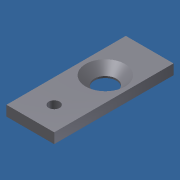
# Autodesk Inventor part: SUPORTE(44)
Saved by Autodesk Inventor 2012 SP1 (Build 160190100, 190)
## iProperties
Created: 2012-07-23
Part Number: SUPORTE(44)
Material: Carbon Steel
Document SubType Name: Modeling
Designer: bruno.silveira
Mass: 11.5689 g
Surface Area: 12.74 cm^2
Volume: 1.47 cm^3
Density: 7.87 g/cm^3
Author: bruno.silveira
Autodesk Inventor part; units mm, degrees
ref_plane "YZ Plane" through (0, 0, 0) normal (1, 0, 0) x (0, 1, 0)
ref_plane "XZ Plane" through (0, 0, 0) normal (0, 1, 0) x (-1, 0, 0)
ref_plane "XY Plane" through (0, 0, 0) normal (0, 0, 1) x (1, 0, 0)
sketch "Sketch1" plane through (0, 0, 0) normal (0, 0, 1) x (1, 0, 0)
  line L0 (0, 0) -> (14, 0)
  line L1 (14, 0) -> (14, 35)
  line L2 (14, 35) -> (0, 35)
  line L3 (0, 35) -> (0, 0)
  dimension "d0" = 14
  dimension "d1" = 35
  constraints: 8 end point, 2 parallel, 1 horizontal, 1 perpendicular
  measures "d0" distance of L1.end L2.end
  measures "d1" distance of L2.end L0.start
extrude "Extrusion1" add sketch "Sketch1" along normal blind 3
sketch "Sketch2" plane through (0, 0, 3) normal (0, 0, 1) x (1, 0, 0)
  line L0 (0, 0) -> (0, 35) projected
  line L1 (0, 35) -> (14, 35) projected
  point P0 (7, 22)
  dimension "d4" = 13
  dimension "d5" = 7
  measures "d4" distance from line of L1 point (7, 22)
  measures "d5" distance from line of L0 point (7, 22)
hole "Hole1" at (7, 22, 3) direction (0, 0, -1) diameter 6.5 depth 3 tip angle 118 countersink diameter 11.5 countersink angle 90
sketch "Sketch3" plane through (0, 0, 0) normal (0, 0, -1) x (-1, 0, 0)
  line L0 (0, 0) -> (-14, 0) projected
  line L1 (0, 35) -> (0, 0) projected
  point P0 (-7, 7)
  dimension "d13" = 7
  dimension "d14" = 7
  measures "d13" distance from line of L0 point (-7, 7)
  measures "d14" distance from line of L1 point (-7, 7)
hole "Hole2" at (7, 7, 0) direction (0, 0, 1) diameter 3.2 depth 3 tip angle 118 countersink diameter 4 countersink angle 90
body "Solid1"
